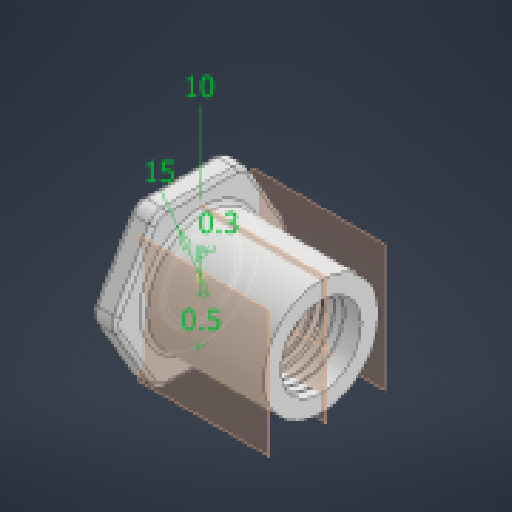
# Autodesk Inventor part: screw_v1
Saved by Autodesk Inventor 2026.1 (Build 301233020, 233B)
## iProperties
Created: 2025-12-01
Part Number: screw_v1
Material: 일반
Document SubType Name: Modeling
Designer: jaewook
Density: 1 g/cm^3
Appearance: 기본값
Author: jaewook
Autodesk Inventor part; units mm, degrees
ref_plane "YZ Plane" through (0, 0, 0) normal (1, 0, 0) x (0, 1, 0)
ref_plane "XZ Plane" through (0, 0, 0) normal (0, 1, 0) x (-1, 0, 0)
sketch "스케치1" plane through (0, 0, 0) normal (1, 0, 0) x (0, 1, 0)
  circle A0 centre (0, 0) radius 5
  circle A1 centre (0, 0) radius 5.3
  circle A2 centre (0, 0) radius 7.5
  circle A3 centre (0, 0) radius 4.5
  dimension "d0" = 10
  dimension "d1" = 0.3
  dimension "d2" = 15
  dimension "d3" = 0.5
  constraints: 4 centre point, 2 coincident
  measures "d0" diameter of A0
  measures "d1" radial gap between concentric circles of A1 A0
  measures "d2" diameter of A2
  measures "d3" radial gap between concentric circles of A0 A3
extrude "돌출1" add sketch "스케치1" along normal blind 15.6 contours A0 | A1 | A2
ref_plane "작업 평면3" through (0, 0, 0) normal (0, 0, 1) x (1, 0, 0)
ref_plane "작업 평면1" through (0, 0, 7.5) normal (0, 0, 1) x (1, 0, 0)
ref_plane "작업 평면2" through (0, 0, -7.5) normal (0, 0, 1) x (1, 0, 0)
sketch "스케치2" plane through (0, 0, 0) normal (0, 0, 1) x (1, 0, 0)
  line L0 (15.6, -4.5) -> (0, -4.5) projected
  line L1 (15.6, 4.5) -> (15.6, -4.5) projected
  line L2 (15.6, 4.5) -> (0, 4.5) projected
  line L3 (-2.625, -4.3647) -> (-1.375, -4.3647)
  line L4 (-1.375, -4.3647) -> (-2, -5.4472)
  line L5 (-2, -5.4472) -> (-2.625, -4.3647)
  line L6 (-2, -5.4472) -> (-2, -4.3647)
  line L7 (-2.5469, -4.5) -> (-1.4531, -4.5)
  line L8 (-2.2005, -5.1) -> (-1.7995, -5.1)
  point P0 (0, 0)
  point P1 (5, 4.5)
  point P2 (5, -4.5)
  point P3 (-2, -4.5)
  dimension "d13" = 1.25
  dimension "d14" = 60
  dimension "d15" = 1.0825
  dimension "d16" = 0.6
  dimension "d17" = 0.1353
  dimension "d18" = 2
  constraints: 12 end point, 4 point on line, 3 horizontal, 2 midpoint, 1 collinear, 1 equal length
  measures "d13" distance of L3.start L3.end
  measures "d14" angle of L4 L5
  measures "d15" distance from line of L4.end L3
  measures "d16" distance between parallel lines of L8 L7
  measures "d17" distance between parallel lines of L7 L3
  measures "d18" distance of L0.end point (-2, -4.5)
sketch "스케치7" plane through (15.6, 0, 0) normal (1, 0, 0) x (0, 0, -1)
  circle A0 centre (0, 0) radius 4.5 projected
  circle A1 centre (0, 0) radius 7.5 projected
  circle A2 centre (0, 0) radius 5.25
  dimension "d51" = 10.5
  constraints: 1 centre point, 1 coincident
  measures "d51" diameter of A2
extrude "돌출7" cut sketch "스케치7" against normal blind 5 contours A2
coil "코일1" sketch "스케치2" operation cut axis through (0, 0, 0) along (1, 0, 0) pitch 1.25 turns 13 hand right contours L7 L6 L8 L5 | L7 L4 L8 L6 | L8 L6 L5 | L8 L4 L6
sketch "스케치3" plane through (0, 0, 0) normal (-1, 0, 0) x (0, 0, 1)
  arc A0 (-3.8369, -2.3512) -> (-1.0505, -4.3757) centre (0, 0) ccw projected
  circle A1 centre (0, 0) radius 7.5 projected
  line L0 (11.547, 0) -> (5.7735, -10)
  line L1 (5.7735, -10) -> (-5.7735, -10)
  line L2 (-5.7735, -10) -> (-11.547, 0)
  line L3 (-11.547, 0) -> (-5.7735, 10)
  line L4 (-5.7735, 10) -> (5.7735, 10)
  line L5 (5.7735, 10) -> (11.547, 0)
  dimension "d38" = 20
  constraints: 12 end point, 1 coincident, 1 horizontal, 17 other
  measures "d38" distance between parallel lines of L1 L4
extrude "돌출3" add sketch "스케치3" along normal blind 3 contours A1 | L0 L1 L2 L3 L4 L5
fillet "모깎기1" radius 2 6 edges at (-1.5, 10, 5.7735) (-1.5, 10, -5.7735) (-1.5, 0, 11.547) (-1.5, -10, 5.7735) (-1.5, -10, -5.7735) (-1.5, 0, -11.547)
fillet "모깎기2" radius 0.5 25 edges at (0, -7.5, 0) (0, 0, -11.2376) (0, -5, -8.6603) (0, -9.7321, -5.6188) (0, -10, 0) (0, -9.7321, 5.6188) (0, -5, 8.6603) (0, 0, 11.2376) (0, 5, 8.6603) (0, 9.7321, 5.6188) (0, 10, 0) (0, 9.7321, -5.6188) (0, 5, -8.6603) (-3, 0, -11.2376) (-3, -5, -8.6603) (-3, -9.7321, -5.6188) (-3, -10, 0) (-3, -9.7321, 5.6188) (-3, -5, 8.6603) (-3, 0, 11.2376) (-3, 5, 8.6603) (-3, 9.7321, 5.6188) (-3, 10, 0) (-3, 9.7321, -5.6188) (-3, 5, -8.6603)
sketch "스케치4" plane through (-3, 0, 0) normal (-1, 0, 0) x (0, 0, 1)
  circle A0 centre (0, 0) radius 2
  dimension "d35" = 4
  constraints: 1 centre point, 1 coincident
  measures "d35" diameter of A0
extrude "돌출4" cut sketch "스케치4" against normal through all
equation "\"d17\" = 0.125 * d15"
